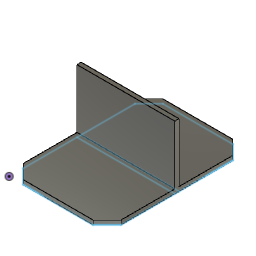
DWST14925 (Autodesk Fusion 360 design; units mm, degrees)
Autodesk Fusion 360 part; units mm, degrees
sketch "Sketch1" plane through (0, 0, 0) normal (0, 0, 1) x (1, 0, 0)
  line L0 (0, 90) -> (10, 100)
  line L1 (70, 90) -> (60, 100)
  line L2 (0, 10) -> (10, 0)
  line L3 (70, 10) -> (60, 0)
  line L4 (10, 100) -> (60, 100)
  line L5 (70, 90) -> (70, 10)
  line L6 (60, 0) -> (10, 0)
  line L7 (0, 10) -> (0, 90)
  line L8 (70, 51.5) -> (0, 51.5)
  line L9 (70, 48.5) -> (0, 48.5)
  constraint perpendicular L4 L5
  constraint perpendicular L5 L6
  constraint perpendicular L6 L7
  constraint coincident L5 L8.start
  constraint coincident L7 L8.end
  constraint perpendicular L7 L8
  constraint coincident L5 L9.start
  constraint coincident L7 L9.end
  constraint perpendicular L7 L9
extrude "Extrude1" add sketch "Sketch1" along normal blind 3 makes body 1
extrude "Extrude2" add sketch "Sketch1" along normal blind 45 separate body contours L5 L7 L8 L9 makes body 2
combine "Combine1" operation add target body 1 tool bodies 2
